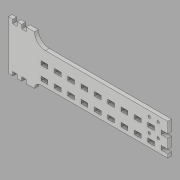
# Autodesk Inventor part: g_arm1
Saved by Autodesk Inventor 2019 (Build 230136000, 136)
## iProperties
Created: 2021-11-01
Part Number: g_arm1
Material: Generic
Document SubType Name: Modeling
Designer: Mohamed
Density: 1 g/cm^3
Appearance: Default
Author: Mohamed
Autodesk Inventor part; units mm, degrees
ref_plane "YZ Plane" through (0, 0, 0) normal (1, 0, 0) x (0, 1, 0)
ref_plane "XZ Plane" through (0, 0, 0) normal (0, 1, 0) x (-1, 0, 0)
ref_plane "XY Plane" through (0, 0, 0) normal (0, 0, 1) x (1, 0, 0)
sketch "Sketch1" plane through (0, 0, 0) normal (0, 0, 1) x (1, 0, 0)
  line L0 (0, 0) -> (250, 0)
  line L1 (250, 0) -> (250, 77)
  line L2 (250, 77) -> (0, 77)
  line L3 (0, 77) -> (0, 0)
  dimension "d0" = 250
  dimension "d1" = 77
  constraints: 8 end point, 2 parallel, 1 horizontal, 1 perpendicular
  measures "d0" distance of L2.end L1.end
  measures "d1" distance of L1.end L0.end
extrude "Extrusion1" add sketch "Sketch1" along normal blind 6
sketch "Sketch2" plane through (0, 0, 6) normal (0, 0, 1) x (1, 0, 0)
  line L0 (250, 77) -> (0, 77) projected
  line L1 (0, 77) -> (7, 77)
  line L2 (7, 77) -> (14, 77)
  line L3 (14, 77) -> (14, 71)
  line L4 (14, 71) -> (7, 71)
  line L5 (7, 71) -> (7, 77)
  line L6 (0, 0) -> (250, 0) projected
  line L7 (0, 0) -> (7, 0)
  line L8 (7, 0) -> (14, 0)
  line L9 (14, 0) -> (14, 6)
  line L10 (14, 6) -> (7, 6)
  line L11 (7, 6) -> (7, 0)
  dimension "d4" = 7
  dimension "d5" = 7
  dimension "d6" = 6
  dimension "d7" = 7
  dimension "d8" = 7
  dimension "d9" = 6
  constraints: 20 end point, 4 parallel, 2 horizontal, 2 perpendicular, 2 point on line
  measures "d4" distance of L0.end L1.end
  measures "d5" distance of L3.end L4.end
  measures "d6" distance of L2.end L3.end
  measures "d7" distance of L6.start L7.end
  measures "d8" distance of L10.end L9.end
  measures "d9" distance of L9.end L8.end
extrude "Extrusion2" cut sketch "Sketch2" against normal blind 6
pattern_linear "Rectangular Pattern1" count 2 spacing 14 along (1, 0, 0) of "Extrusion2"
sketch "Sketch3" plane through (0, 0, 6) normal (0, 0, 1) x (1, 0, 0)
  line L0 (250, 77) -> (28, 77) projected
  line L1 (41, 77) -> (49.5, 77)
  line L2 (28, 0) -> (250, 0) projected
  line L3 (41, 0) -> (51, 0)
  arc A0 (51, 10) -> (41, 0) centre (51, 0) ccw
  line L4 (41, 77) -> (58, 77)
  arc A1 (41, 77) -> (58, 60) centre (58, 77) ccw
  line L5 (58, 60) -> (250, 60)
  line L6 (51, 10) -> (250, 10)
  line L7 (250, 0) -> (250, 77) projected
  point P0 (0, 0)
  point P1 (0, 77)
  dimension "d15" = 41
  dimension "d21" = 34
  constraints: 10 end point, 6 point on line, 4 point on circle, 2 centre point, 2 coincident, 2 horizontal
  measures "d15" distance of point (0, 77) L1.start
  measures "d21" diameter of A1
extrude "Extrusion3" cut sketch "Sketch3" against normal blind 6
sketch "Sketch4" plane through (0, 0, 6) normal (0, 0, 1) x (1, 0, 0)
  line L0 (28, 0) -> (41, 0) projected
  line L1 (51.45, 16) -> (61.9, 16)
  line L2 (61.9, 16) -> (61.9, 22)
  line L3 (61.9, 22) -> (51.45, 22)
  line L4 (51.45, 22) -> (51.45, 16)
  line L5 (51.45, 37) -> (61.9, 37)
  line L6 (61.9, 37) -> (61.9, 43)
  line L7 (61.9, 43) -> (51.45, 43)
  line L8 (51.45, 43) -> (51.45, 37)
  point P0 (0, 0)
  point P1 (51, 10)
  dimension "d26" = 10.45
  dimension "d27" = 6
  dimension "d28" = 15
  dimension "d29" = 10.45
  dimension "d30" = 6
  constraints: 16 end point, 4 parallel, 2 horizontal, 2 perpendicular
  measures "d26" distance of L3.end L2.end
  measures "d27" distance of L2.end L1.end
  measures "d28" distance of L3.end L5.start
  measures "d29" distance of L7.end L6.end
  measures "d30" distance of L6.end L5.end
extrude "Extrusion4" cut sketch "Sketch4" against normal blind 6
pattern_linear "Rectangular Pattern2" count 10 spacing 20.9 along (1, 0, 0) of "Extrusion4"
sketch "Sketch5" plane through (0, 0, 6) normal (0, 0, 1) x (1, 0, 0)
  line L0 (250, 43) -> (250, 60) projected
  circle A0 centre (235, 51.5) radius 2
  circle A1 centre (221, 51.5) radius 2
  line L1 (250, 22) -> (250, 37) projected
  circle A2 centre (221, 29.5) radius 2
  circle A3 centre (235, 29.5) radius 2
  point P0 (0, 0)
  dimension "d37" = 4
  dimension "d39" = 4
  dimension "d40" = 4
  dimension "d41" = 4
  constraints: 4 centre point
  measures "d37" diameter of A0
  measures "d39" diameter of A1
  measures "d40" diameter of A2
  measures "d41" diameter of A3
extrude "Extrusion5" cut sketch "Sketch5" against normal blind 6
body "Solid1"
